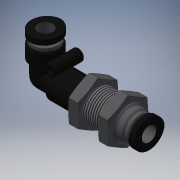
# Autodesk Inventor part: ElbowBulkhead(0.25inOD)-1111-2017
Saved by Autodesk Inventor 2016 SP2 (Build 200236200, 236)
## iProperties
Category: PARTsolutions
Company: BIMBA
Created: 2017-03-17
Part Number: ElbowBulkhead(0.25inOD)-1111-2017
Catalog Web Link: www.cadenas.de
Description: CPEUB-Elbow Bulkhead
Vendor: BIMBA
Document SubType Name: Modeling
Designer: psAdmin
Manufacturer: BIMBA
Mass: 7.12352 g
Surface Area: 50.5168 cm^2
Volume: 7.12352 cm^3
Density: 1 g/cm^3
Material: Generic
Appearance: PSOLRGB-175-175-175
PSOL_IDENT_0: {$CADENAS_DATA\23d-libs\bimba\pneumadyne\fittings\push_to_connect\elbow_bulkhead.prj},157 {VTYP=3D},
PSOL_IDENT_1: {NB=CPEUB250},{LINA=CPEUB250},{NN=CPEUB},{DATE=27.02.2017 06:59:47},{GEOMDATE=20.06.2014 12:01:00},{
PSOL_IDENT_2: VERSION=},{LINEID=20},{LINESUBID=-1},{WBVAR=}  {NB=CPEUB250},{LINA=CPEUB250},{KT=DUMMY},{PN=CPEUB250
PSOL_IDENT_3: },{D=0.25000000},{DPN=250},{E=0.7},{B=1.8},{P=0.5},{A=0.3},{M=M14},{MND=14},{H=0.68750000},{QTY=5},{
PSOL_IDENT_4: PITCH=1},{CMAJ=0.538},{CMIN=0.4875}
NN: CPEUB
NT: Elbow Bulkhead
NB: CPEUB250
NBSYN: $PN.
LINA: CPEUB250
PN: CPEUB250
D: 1/4
E: 0.7
B: 1.8
P: 0.5
M: M14
H: 11/16
QTY: 5
SUPPLIER: BIMBA
ARTICLENO: CPEUB250
BOMINFO: CPEUB250
CREATOR: CADENAS GmbH
Title: CPEUB250
Author: Cadenas PARTsolutions
Comments: Elbow Bulkhead
Autodesk Inventor part; units mm, degrees
sketch "Sketch_1" plane through (0, 0, 0) normal (0, 0, 1) x (1, 0, 0)
  line L0 (0, -5.08) -> (0, 17.78)
  line L1 (0, 17.78) -> (5.8928, 17.78)
  arc A0 (6.35, 17.3228) -> (5.8928, 17.78) centre (5.8928, 17.3228) ccw
  line L2 (6.35, 17.3228) -> (6.35, 15.494)
  line L3 (6.35, 15.494) -> (4.445, 15.494)
  line L4 (4.445, 15.494) -> (4.445, 14.0716)
  line L5 (4.445, 14.0716) -> (5.4864, 14.0716)
  arc A1 (5.715, 13.843) -> (5.4864, 14.0716) centre (5.4864, 13.843) ccw
  line L6 (5.715, 13.843) -> (5.715, 12.7)
  line L7 (5.715, 12.7) -> (6.35, 12.065)
  line L8 (6.35, 12.065) -> (6.35, 6.4135)
  line L9 (6.35, 6.4135) -> (5.08, 5.3478)
  line L10 (5.08, 5.3478) -> (5.08, 0)
  arc A2 (0, -5.08) -> (5.08, 0) centre (0, 0) ccw
  line L11 (0, -5.08) -> (0, 17.78)
  constraints: 24 end point, 6 point on circle, 3 centre point
revolve "Revolution1" add sketch "Sketch_1" angle 360 about axis through (0, -5.08, 0) along (0, -1, 0)
sketch "Sketch_2" plane through (0, 0, 0) normal (0, 0, 1) x (1, 0, 0)
  line L0 (45.72, 0) -> (-5.08, 0)
  line L1 (-5.08, 0) -> (0, 5.08)
  line L2 (0, 5.08) -> (5.3478, 5.08)
  line L3 (5.3478, 5.08) -> (6.4135, 6.35)
  line L4 (6.4135, 6.35) -> (17.145, 6.35)
  line L5 (17.145, 6.35) -> (17.78, 5.715)
  line L6 (17.78, 5.715) -> (17.78, 6.3865)
  line L7 (17.78, 6.3865) -> (18.3935, 7)
  line L8 (18.3935, 7) -> (37.1055, 7)
  line L9 (37.1055, 7) -> (37.719, 6.3865)
  line L10 (37.719, 6.3865) -> (37.719, 6.35)
  line L11 (37.719, 6.35) -> (40.005, 6.35)
  line L12 (40.005, 6.35) -> (40.64, 5.715)
  line L13 (40.64, 5.715) -> (41.783, 5.715)
  arc A0 (42.0116, 5.4864) -> (41.783, 5.715) centre (41.783, 5.4864) ccw
  line L14 (42.0116, 5.4864) -> (42.0116, 4.445)
  line L15 (42.0116, 4.445) -> (43.434, 4.445)
  line L16 (43.434, 4.445) -> (43.434, 6.35)
  line L17 (43.434, 6.35) -> (45.2628, 6.35)
  arc A1 (45.72, 5.8928) -> (45.2628, 6.35) centre (45.2628, 5.8928) ccw
  line L18 (45.72, 5.8928) -> (45.72, 0)
  line L19 (45.72, 0) -> (-5.08, 0)
  constraints: 40 end point, 4 point on circle, 2 centre point
revolve "Revolution2" add sketch "Sketch_2" angle 360 about axis through (45.72, 0, 0) along (1, 0, 0)
thread "Thread1" size "M14x1" class "6g" standard "ISO Metric profile" full length
sketch "Sketch_6" plane through (0, 0, 0) normal (0, 0, 1) x (1, 0, 0)
  line L0 (36.576, 0) -> (0, 0)
  line L1 (0, 0) -> (0, 3.175)
  line L2 (0, 3.175) -> (18.796, 3.175)
  line L3 (18.796, 3.175) -> (18.796, 8.7312)
  line L4 (18.796, 8.7312) -> (19.2639, 10.4775)
  line L5 (19.2639, 10.4775) -> (22.9001, 10.4775)
  line L6 (22.9001, 10.4775) -> (23.368, 8.7312)
  line L7 (23.368, 8.7312) -> (23.368, 7)
  line L8 (23.368, 7) -> (32.004, 7)
  line L9 (32.004, 7) -> (32.004, 8.7312)
  line L10 (32.004, 8.7312) -> (32.4719, 10.4775)
  line L11 (32.4719, 10.4775) -> (36.1081, 10.4775)
  line L12 (36.1081, 10.4775) -> (36.576, 8.7312)
  line L13 (36.576, 8.7312) -> (36.576, 0)
  line L14 (36.576, 0) -> (0, 0)
  constraints: 30 end point
revolve "Revolution3" add sketch "Sketch_6" angle 360 about axis through (36.576, 0, 0) along (1, 0, 0)
sketch "Sketch_3" plane through (8.255, 0, 0) normal (1, 0, 0) x (0, 0, -1)
  line L0 (6.35, 8.5725) -> (-6.35, 8.5725)
  line L1 (-6.35, 9.8425) -> (6.35, 9.8425)
  line L2 (6.35, 9.8425) -> (6.35, 10.795)
  arc A0 (6.35, 10.795) -> (6.0325, 11.1125) centre (6.0325, 10.795) ccw
  line L3 (6.0325, 11.1125) -> (-6.0325, 11.1125)
  arc A1 (-6.0325, 11.1125) -> (-6.35, 10.795) centre (-6.0325, 10.795) ccw
  line L4 (-6.35, 10.795) -> (-6.35, 9.8425)
  constraints: 10 end point, 4 point on circle, 2 centre point
revolve "Revolution4" add sketch "Sketch_3" angle 360 about axis through (8.255, 8.5725, -6.35) along (0, 0, -1)
sketch "Sketch_4" plane through (0, 0, 0) normal (0, 0, 1) x (1, 0, 0)
  line L0 (0, -1.5875) -> (0, 17.78)
  line L1 (0, 17.78) -> (3.175, 17.78)
  line L2 (3.175, 17.78) -> (3.175, 4.445)
  line L3 (3.175, 4.445) -> (1.5875, 4.445)
  line L4 (1.5875, 4.445) -> (1.5875, 0)
  arc A0 (0, -1.5875) -> (1.5875, 0) centre (0, 0) ccw
  line L5 (0, -1.5875) -> (0, 17.78)
  constraints: 12 end point, 2 point on circle, 1 centre point
revolve "Revolution5" cut sketch "Sketch_4" angle 360 about axis through (0, -1.5875, 0) along (0, -1, 0)
sketch "Sketch6" plane through (45.72, 0, 0) normal (1, 0, 0) x (0, 0, -1)
  point P0 (0, 0)
hole "Hole1" at (45.72, 0, 0) direction (-1, 0, 0) diameter 3.175 depth 45.72 counterbore diameter 6.35 counterbore depth 41.275
sketch "Sketch_7" plane through (36.576, 0, 0) normal (1, 0, 0) x (0, 0, -1)
  line L0 (-17.4625, -10.082) -> (0, -20.164)
  line L1 (0, -20.164) -> (17.4625, -10.082)
  line L2 (17.4625, -10.082) -> (17.4625, 10.082)
  line L3 (17.4625, 10.082) -> (0, 20.164)
  line L4 (0, 20.164) -> (-17.4625, 10.082)
  line L5 (-17.4625, 10.082) -> (-17.4625, -10.082)
  line L6 (-8.7312, -5.041) -> (0, -10.082)
  line L7 (0, -10.082) -> (8.7312, -5.041)
  line L8 (8.7312, -5.041) -> (8.7312, 5.041)
  line L9 (8.7312, 5.041) -> (0, 10.082)
  line L10 (0, 10.082) -> (-8.7312, 5.041)
  line L11 (-8.7312, 5.041) -> (-8.7312, -5.041)
  constraints: 24 end point
extrude "Extrusion1" cut sketch "Sketch_7" against normal blind 22.86
sketch "Sketch_10" plane through (0, 0, 0) normal (0, 0, 1) x (1, 0, 0)
  line L0 (-6.35, 15.494) -> (43.434, 15.494)
  line L1 (43.434, 15.494) -> (43.434, -6.35)
  line L2 (43.434, -6.35) -> (45.72, -6.35)
  line L3 (45.72, -6.35) -> (45.72, 17.78)
  line L4 (45.72, 17.78) -> (-6.35, 17.78)
  line L5 (-6.35, 17.78) -> (-6.35, 15.494)
  constraints: 12 end point
extrude "Extrusion2" cut sketch "Sketch_10" along normal mid plane 12.7
sketch "Sketch_11" plane through (45.72, 0, 0) normal (1, 0, 0) x (0, 0, -1)
  arc A0 (-6.3383, 2.0638) -> (-6.3383, -2.0638) centre (-2.2775, 0) ccw
  arc A1 (-6.3383, -2.0638) -> (6.3383, -2.0638) centre (0, 0.7391) ccw
  arc A2 (6.3383, -2.0638) -> (6.3383, 2.0638) centre (2.2775, 0) ccw
  arc A3 (6.3383, 2.0638) -> (-6.3383, 2.0638) centre (0, -0.7391) ccw
  circle A4 centre (0, 0) radius 3.175
  constraints: 8 point on circle, 5 centre point
extrude "Extrusion3" add sketch "Sketch_11" against normal blind 2.286
sketch "Sketch_12" plane through (0, 17.78, 0) normal (0, 1, 0) x (1, 0, 0)
  arc A0 (-2.0638, 6.3383) -> (-2.0638, -6.3383) centre (0.7391, 0) ccw
  arc A1 (-2.0638, -6.3383) -> (2.0638, -6.3383) centre (0, -2.2775) ccw
  arc A2 (2.0638, -6.3383) -> (2.0638, 6.3383) centre (-0.7391, 0) ccw
  arc A3 (2.0638, 6.3383) -> (-2.0638, 6.3383) centre (0, 2.2775) ccw
  circle A4 centre (0, 0) radius 3.175
  constraints: 8 point on circle, 5 centre point
extrude "Extrusion4" add sketch "Sketch_12" against normal blind 2.286
ref_plane "b1_XY" through (0, 0, 0) normal (0, 0, 1) x (1, 0, 0)
ref_plane "b1_YZ" through (0, 0, 0) normal (1, 0, 0) x (0, 1, 0)
ref_plane "b1_ZX" through (0, 0, 0) normal (0, 1, 0) x (0, 0, 1)
ref_plane "b2_XY" through (45.72, 0, 0) normal (0, 0, 1) x (1, 0, 0)
ref_plane "b2_YZ" through (45.72, 0, 0) normal (1, 0, 0) x (0, 1, 0)
ref_plane "b2_ZX" through (45.72, 0, 0) normal (0, 1, 0) x (0, 0, 1)
ref_plane "d1_XY" through (45.72, 3.175, 0) normal (0, 0, 1) x (1, 0, 0)
ref_plane "d1_YZ" through (45.72, 3.175, 0) normal (1, 0, 0) x (0, 1, 0)
ref_plane "d1_ZX" through (45.72, 3.175, 0) normal (0, 1, 0) x (0, 0, 1)
ref_plane "d2_XY" through (45.72, -3.175, 0) normal (0, 0, 1) x (1, 0, 0)
ref_plane "d2_YZ" through (45.72, -3.175, 0) normal (1, 0, 0) x (0, 1, 0)
ref_plane "d2_ZX" through (45.72, -3.175, 0) normal (0, 1, 0) x (0, 0, 1)
ref_plane "dd1_XY" through (-3.175, 17.78, 0) normal (0, 0, 1) x (1, 0, 0)
ref_plane "dd1_YZ" through (-3.175, 17.78, 0) normal (1, 0, 0) x (0, 1, 0)
ref_plane "dd1_ZX" through (-3.175, 17.78, 0) normal (0, 1, 0) x (0, 0, 1)
ref_plane "dd2_XY" through (3.175, 17.78, 0) normal (0, 0, 1) x (1, 0, 0)
ref_plane "dd2_YZ" through (3.175, 17.78, 0) normal (1, 0, 0) x (0, 1, 0)
ref_plane "dd2_ZX" through (3.175, 17.78, 0) normal (0, 1, 0) x (0, 0, 1)
ref_plane "e1_XY" through (0, 17.78, 0) normal (0, 0, 1) x (1, 0, 0)
ref_plane "e1_YZ" through (0, 17.78, 0) normal (1, 0, 0) x (0, 1, 0)
ref_plane "e1_ZX" through (0, 17.78, 0) normal (0, 1, 0) x (0, 0, 1)
ref_plane "h1_XY" through (36.576, 0, 8.7312) normal (1, 0, 0) x (0, 0, -1)
ref_plane "h1_YZ" through (36.576, 0, 8.7312) normal (0, 0, -1) x (0, 1, 0)
ref_plane "h1_ZX" through (36.576, 0, 8.7312) normal (0, 1, 0) x (1, 0, 0)
ref_plane "h2_XY" through (36.576, 0, -8.7312) normal (1, 0, 0) x (0, 0, -1)
ref_plane "h2_YZ" through (36.576, 0, -8.7312) normal (0, 0, -1) x (0, 1, 0)
ref_plane "h2_ZX" through (36.576, 0, -8.7312) normal (0, 1, 0) x (1, 0, 0)
ref_plane "m1_XY" through (36.576, 7, 0) normal (0, 0, 1) x (1, 0, 0)
ref_plane "m1_YZ" through (36.576, 7, 0) normal (1, 0, 0) x (0, 1, 0)
ref_plane "m1_ZX" through (36.576, 7, 0) normal (0, 1, 0) x (0, 0, 1)
ref_plane "m2_XY" through (36.576, -7, 0) normal (0, 0, 1) x (1, 0, 0)
ref_plane "m2_YZ" through (36.576, -7, 0) normal (1, 0, 0) x (0, 1, 0)
ref_plane "m2_ZX" through (36.576, -7, 0) normal (0, 1, 0) x (0, 0, 1)
ref_plane "p1_XY" through (-6.35, 12.065, 0) normal (0, 0, 1) x (1, 0, 0)
ref_plane "p1_YZ" through (-6.35, 12.065, 0) normal (1, 0, 0) x (0, 1, 0)
ref_plane "p1_ZX" through (-6.35, 12.065, 0) normal (0, 1, 0) x (0, 0, 1)
ref_plane "p2_XY" through (6.35, 12.065, 0) normal (0, 0, 1) x (1, 0, 0)
ref_plane "p2_YZ" through (6.35, 12.065, 0) normal (1, 0, 0) x (0, 1, 0)
ref_plane "p2_ZX" through (6.35, 12.065, 0) normal (0, 1, 0) x (0, 0, 1)
body "Solid1"
